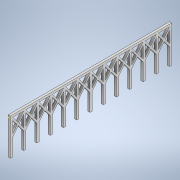
# Autodesk Inventor part: platform part
Saved by Autodesk Inventor 2021 (Build 250183000, 183)
## iProperties
Created: 2021-04-19
Part Number: platform part
Material: Generic
Document SubType Name: Modeling
Designer: miw14
Density: 1 g/cm^3
Appearance: Default
Author: miw14
Autodesk Inventor part; units mm, degrees
ref_plane "YZ Plane" through (0, 0, 0) normal (1, 0, 0) x (0, 1, 0)
ref_plane "XZ Plane" through (0, 0, 0) normal (0, 1, 0) x (-1, 0, 0)
ref_plane "XY Plane" through (0, 0, 0) normal (0, 0, 1) x (1, 0, 0)
sketch "Sketch1" plane through (0, 0, 0) normal (1, 0, 0) x (0, 1, 0)
  line L0 (0, 0) -> (254, 0)
  line L1 (254, 0) -> (254, -18288)
  line L2 (254, -18288) -> (0, -18288)
  line L3 (0, -18288) -> (0, 0)
  line L4 (0, 0) -> (-3962.4, 0)
  line L5 (-3962.4, 0) -> (-3962.4, -254)
  line L6 (-3962.4, -254) -> (0, -254)
  line L7 (0, -254) -> (0, 0)
  line L8 (-3962.4, -1778) -> (0, -1778)
  line L9 (-3962.4, -1524) -> (-3962.4, -1778)
  line L10 (0, -1524) -> (-3962.4, -1524)
  line L11 (-3962.4, -3302) -> (0, -3302)
  line L12 (-3962.4, -3048) -> (-3962.4, -3302)
  line L13 (0, -3048) -> (-3962.4, -3048)
  line L14 (-3962.4, -4826) -> (0, -4826)
  line L15 (-3962.4, -4572) -> (-3962.4, -4826)
  line L16 (0, -4572) -> (-3962.4, -4572)
  line L17 (-3962.4, -6350) -> (0, -6350)
  line L18 (-3962.4, -6096) -> (-3962.4, -6350)
  line L19 (0, -6096) -> (-3962.4, -6096)
  line L20 (-3962.4, -7874) -> (0, -7874)
  line L21 (-3962.4, -7620) -> (-3962.4, -7874)
  line L22 (0, -7620) -> (-3962.4, -7620)
  line L23 (-3962.4, -9398) -> (0, -9398)
  line L24 (-3962.4, -9144) -> (-3962.4, -9398)
  line L25 (0, -9144) -> (-3962.4, -9144)
  line L26 (-3962.4, -10922) -> (0, -10922)
  line L27 (-3962.4, -10668) -> (-3962.4, -10922)
  line L28 (0, -10668) -> (-3962.4, -10668)
  line L29 (-3962.4, -12446) -> (0, -12446)
  line L30 (-3962.4, -12192) -> (-3962.4, -12446)
  line L31 (0, -12192) -> (-3962.4, -12192)
  line L32 (-3962.4, -13970) -> (0, -13970)
  line L33 (-3962.4, -13716) -> (-3962.4, -13970)
  line L34 (0, -13716) -> (-3962.4, -13716)
  line L35 (-3962.4, -15494) -> (0, -15494)
  line L36 (-3962.4, -15240) -> (-3962.4, -15494)
  line L37 (0, -15240) -> (-3962.4, -15240)
  line L38 (-3962.4, -17018) -> (0, -17018)
  line L39 (-3962.4, -16764) -> (-3962.4, -17018)
  line L40 (0, -16764) -> (-3962.4, -16764)
  line L41 (0, -254) -> (-1674.3057, -1524)
  line L42 (-1981.2, -1524) -> (-306.8943, -254)
  line L43 (0, -1524) -> (-1625.7095, -254)
  line L44 (-1981.2, -254) -> (-355.4905, -1524)
  line L45 (-1981.2, -1778) -> (-355.4905, -3048)
  line L46 (0, -3048) -> (-1625.7095, -1778)
  line L47 (0, -1778) -> (-1674.3057, -3048)
  line L48 (-1981.2, -3048) -> (-306.8943, -1778)
  line L49 (-1981.2, -3302) -> (-355.4905, -4572)
  line L50 (0, -4572) -> (-1625.7095, -3302)
  line L51 (0, -3302) -> (-1674.3057, -4572)
  line L52 (-1981.2, -4572) -> (-306.8943, -3302)
  line L53 (-1981.2, -4826) -> (-355.4905, -6096)
  line L54 (0, -6096) -> (-1625.7095, -4826)
  line L55 (0, -4826) -> (-1674.3057, -6096)
  line L56 (-1981.2, -6096) -> (-306.8943, -4826)
  line L57 (-1981.2, -6350) -> (-355.4905, -7620)
  line L58 (0, -7620) -> (-1625.7095, -6350)
  line L59 (0, -6350) -> (-1674.3057, -7620)
  line L60 (-1981.2, -7620) -> (-306.8943, -6350)
  line L61 (-1981.2, -7874) -> (-355.4905, -9144)
  line L62 (0, -9144) -> (-1625.7095, -7874)
  line L63 (0, -7874) -> (-1674.3057, -9144)
  line L64 (-1981.2, -9144) -> (-306.8943, -7874)
  line L65 (-1981.2, -9398) -> (-355.4905, -10668)
  line L66 (0, -10668) -> (-1625.7095, -9398)
  line L67 (0, -9398) -> (-1674.3057, -10668)
  line L68 (-1981.2, -10668) -> (-306.8943, -9398)
  line L69 (-1981.2, -10922) -> (-355.4905, -12192)
  line L70 (0, -12192) -> (-1625.7095, -10922)
  line L71 (0, -10922) -> (-1674.3057, -12192)
  line L72 (-1981.2, -12192) -> (-306.8943, -10922)
  line L73 (-1981.2, -12446) -> (-355.4905, -13716)
  line L74 (0, -13716) -> (-1625.7095, -12446)
  line L75 (0, -12446) -> (-1674.3057, -13716)
  line L76 (-1981.2, -13716) -> (-306.8943, -12446)
  line L77 (-1981.2, -13970) -> (-355.4905, -15240)
  line L78 (0, -15240) -> (-1625.7095, -13970)
  line L79 (0, -13970) -> (-1674.3057, -15240)
  line L80 (-1981.2, -15240) -> (-306.8943, -13970)
  line L81 (-1981.2, -15494) -> (-355.4905, -16764)
  line L82 (0, -16764) -> (-1625.7095, -15494)
  line L83 (0, -15494) -> (-1674.3057, -16764)
  line L84 (-1981.2, -16764) -> (-306.8943, -15494)
  line L85 (-1981.2, -17018) -> (-355.4905, -18288)
  line L86 (0, -18288) -> (-1625.7095, -17018)
  line L87 (0, -17018) -> (-1674.3057, -18288)
  line L88 (-1981.2, -18288) -> (-306.8943, -17018)
  line L89 (254, -18288) -> (-3962.4, -18288)
  line L90 (-3962.4, -18288) -> (-3962.4, -18542)
  line L91 (-3962.4, -18542) -> (254, -18542)
  line L92 (254, -18542) -> (254, -18288)
  point P0 (-824.8249, -879.6489)
  point P1 (0, -254)
  point P2 (-1005.1876, -1016.4583)
  point P3 (-1156.3751, -898.3511)
  point P4 (-1156.3751, -2422.3511)
  point P5 (-1156.3751, -3946.3511)
  point P6 (-1156.3751, -5470.3511)
  point P7 (-1156.3751, -6994.3511)
  point P8 (-1156.3751, -8518.3511)
  point P9 (-1156.3751, -10042.3511)
  point P10 (-1156.3751, -11566.3511)
  point P11 (-1156.3751, -13090.3511)
  point P12 (-1156.3751, -14614.3511)
  point P13 (-1156.3751, -16138.3511)
  point P14 (-1156.3751, -17662.3511)
  point P15 (-976.0124, -2285.5417)
  point P16 (-1005.1876, -2540.4583)
  point P17 (-824.8249, -2403.6489)
  point P18 (0, -1778)
  point P19 (-1005.1876, -17780.4583)
  point P20 (-976.0124, -16001.5417)
  point P21 (-824.8249, -17643.6489)
  point P22 (0, -17018)
  point P23 (-976.0124, -17525.5417)
  point P24 (-976.0124, -14477.5417)
  point P25 (-1005.1876, -16256.4583)
  point P26 (-824.8249, -16119.6489)
  point P27 (0, -15494)
  point P28 (-976.0124, -12953.5417)
  point P29 (-1005.1876, -14732.4583)
  point P30 (-824.8249, -14595.6489)
  point P31 (0, -13970)
  point P32 (-976.0124, -11429.5417)
  point P33 (-1005.1876, -13208.4583)
  point P34 (-824.8249, -13071.6489)
  point P35 (0, -12446)
  point P36 (-976.0124, -9905.5417)
  point P37 (-1005.1876, -11684.4583)
  point P38 (-824.8249, -11547.6489)
  point P39 (0, -10922)
  point P40 (-976.0124, -8381.5417)
  point P41 (-1005.1876, -10160.4583)
  point P42 (-824.8249, -10023.6489)
  point P43 (0, -9398)
  point P44 (-976.0124, -6857.5417)
  point P45 (-1005.1876, -8636.4583)
  point P46 (-824.8249, -8499.6489)
  point P47 (0, -7874)
  point P48 (-976.0124, -5333.5417)
  point P49 (-1005.1876, -7112.4583)
  point P50 (-824.8249, -6975.6489)
  point P51 (0, -6350)
  point P52 (-1005.1876, -5588.4583)
  point P53 (-824.8249, -5451.6489)
  point P54 (0, -4826)
  point P55 (-976.0124, -3809.5417)
  point P56 (-1005.1876, -4064.4583)
  point P57 (-824.8249, -3927.6489)
  point P58 (0, -3302)
  point P59 (-976.0124, -761.5417)
  dimension "d0" = 18288
  dimension "d1" = 254
  dimension "d2" = 3962.4
  dimension "d3" = 254
  dimension "d6" = 1524
  dimension "d13" = 1524
  dimension "d18" = 254
  constraints: 184 end point, 132 vertical alignment, 73 parallel, 11 collinear, 4 point on line, 3 horizontal, 3 perpendicular, 2 midpoint, 1 vertical, 3 other
  measures "d0" distance of L0.end L1.end
  measures "d1" distance of L1.end L2.end
  measures "d2" distance of L5.end L6.end
  measures "d3" distance of L4.end L5.end
  measures "d6" distance of L5.end L8.start
  measures "d13" distance of L44.start L45.start
  measures "d18" distance of L89.end L90.end
extrude "Extrusion1" add sketch "Sketch1" along normal blind 254 contours L0 L1 L2 L3 | L3 L6 L5 L4 | L41 L43 L42 L6 | L92 L91 L90 L89 L2 | L3 L8 L9 L10 | L10 L44 L41 L43 | L41 L44 L42 L43 | L89 L85 L87 L86 | L47 L46 L48 L8 | L43 L42 L44 L6 | L41 L10 L42 L44 | L38 L39 L40 L3 | L87 L86 L88 L38 | L87 L85 L88 L86 | L3 L11 L12 L13 | L13 L45 L47 L46 | L47 L45 L48 L46 | L40 L81 L83 L82 | L88 L85 L38 L86 | L87 L89 L88 L85 | L51 L50 L52 L11 | L46 L48 L45 L8 | L47 L13 L48 L45 | L35 L36 L37 L3 | L83 L82 L84 L35 | L83 L81 L84 L82 | L3 L14 L15 L16 | L16 L49 L51 L50 | L51 L49 L52 L50 | L37 L77 L79 L78 | L40 L84 L81 L83 | L84 L81 L35 L82 | L55 L54 L56 L14 | L50 L52 L49 L11 | L51 L16 L52 L49 | L32 L33 L34 L3 | L79 L78 L80 L32 | L79 L77 L80 L78 | L3 L17 L18 L19 | L19 L53 L55 L54 | L55 L53 L56 L54 | L34 L73 L75 L74 | L37 L80 L77 L79 | L80 L77 L32 L78 | L59 L58 L60 L17 | L54 L56 L53 L14 | L55 L19 L56 L53 | L29 L30 L31 L3 | L75 L74 L76 L29 | L75 L73 L76 L74 | L3 L20 L21 L22 | L22 L57 L59 L58 | L59 L57 L60 L58 | L31 L69 L71 L70 | L34 L76 L73 L75 | L76 L73 L29 L74 | L63 L62 L64 L20 | L58 L60 L57 L17 | L59 L22 L60 L57 | L26 L27 L28 L3 | L71 L70 L72 L26 | L71 L69 L72 L70 | L3 L23 L24 L25 | L25 L61 L63 L62 | L63 L61 L64 L62 | L28 L65 L67 L66 | L31 L72 L69 L71 | L72 L69 L26 L70 | L67 L66 L68 L23 | L62 L64 L61 L20 | L63 L25 L64 L61 | L67 L65 L68 L66 | L28 L68 L65 L67 | L68 L65 L23 L66
sketch "Sketch2" plane through (0, -3962.4, 0) normal (0, 0, 1) x (1, 0, 0)
  point P0 (0, 3962.4)
body "Solid1"
